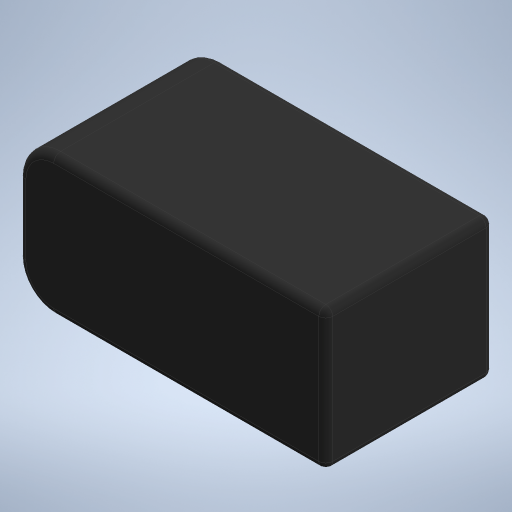
# Autodesk Inventor part: baterie
Saved by Autodesk Inventor 2023 (Build 270158000, 158)
## iProperties
Created: 2023-03-20
Part Number: baterie
Material: Všeobecné
Document SubType Name: Modeling
Designer: Simak
Density: 1 g/cm^3
Appearance: Výchozí
Author: Simak
Autodesk Inventor part; units mm, degrees
ref_plane "YZ Plane" through (0, 0, 0) normal (1, 0, 0) x (0, 1, 0)
ref_plane "XZ Plane" through (0, 0, 0) normal (0, 1, 0) x (-1, 0, 0)
ref_plane "XY Plane" through (0, 0, 0) normal (0, 0, 1) x (1, 0, 0)
sketch "Náčrt1" plane through (0, 0, 0) normal (0, 0, 1) x (1, 0, 0)
  line L0 (0, 0) -> (44, 0)
  line L1 (44, 0) -> (44, 20)
  line L2 (44, 20) -> (0, 20)
  line L3 (0, 20) -> (0, 0)
  dimension "d0" = 44
  dimension "d1" = 20
  constraints: 8 end point, 2 parallel, 1 horizontal, 1 perpendicular
  measures "d0" distance of L2.end L1.end
  measures "d1" distance of L0.end L1.end
extrude "Vysunutí1" add sketch "Náčrt1" along normal blind 24
fillet "Zaoblení1" radius 5 2 edges at (0, 20, 12) (0, 0, 12)
fillet "Zaoblení2" radius 1 14 edges at (1.4645, 18.5355, 0) (0, 10, 0) (1.4645, 1.4645, 0) (24.5, 0, 0) (24.5, 20, 0) (44, 10, 0) (44, 20, 12) (44, 0, 12) (44, 10, 24) (1.4645, 1.4645, 24) (0, 10, 24) (1.4645, 18.5355, 24) (24.5, 20, 24) (24.5, 0, 24)
